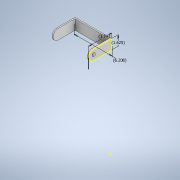
# Autodesk Inventor part: small side peice
Saved by Autodesk Inventor 2021 (Build 250183000, 183)
## iProperties
Created: 2021-08-21
Part Number: small side peice
Material: Generic
Document SubType Name: Modeling
Designer: newic
Density: 1 g/cm^3
Appearance: Default
Author: newic
Autodesk Inventor part; units mm, degrees
ref_plane "YZ Plane" through (0, 0, 0) normal (1, 0, 0) x (0, 1, 0)
ref_plane "XZ Plane" through (0, 0, 0) normal (0, 1, 0) x (-1, 0, 0)
ref_plane "XY Plane" through (0, 0, 0) normal (0, 0, 1) x (1, 0, 0)
sketch "Sketch1" plane through (0, 0, 0) normal (1, 0, 0) x (0, 1, 0)
  line L0 (920.75, 0) -> (0, 0)
  line L1 (0, 0) -> (920.75, 0)
  line L2 (-297.6389, 409.8513) -> (2710.7909, 409.8513) construction
  line L3 (2710.7909, 409.8513) -> (2710.7909, -1716.9746) construction
  line L4 (2710.7909, -1716.9746) -> (-297.6389, -1716.9746) construction
  line L5 (-297.6389, -1716.9746) -> (-297.6389, 409.8513) construction
  line L6 (0, 0) -> (920.75, 0)
  line L7 (920.75, 0) -> (920.75, 100.33)
  line L8 (0, 100.33) -> (920.75, 100.33)
  line L9 (0, 0) -> (0, 100.33)
  line L10 (0, 100.33) -> (0, 120.65)
  line L11 (0, 120.65) -> (920.75, 120.65)
  line L12 (920.75, 120.65) -> (920.75, 100.33)
  line L13 (0, 120.65) -> (0, 196.85)
  line L14 (920.75, 196.85) -> (920.75, 120.65)
  line L15 (477.9962, 0) -> (477.9962, -13.97)
  line L16 (477.9962, -13.97) -> (434.8162, -13.97)
  line L17 (434.8162, -13.97) -> (434.8162, 0)
  line L18 (133.294, 0) -> (133.294, -13.97)
  line L19 (133.294, -13.97) -> (90.114, -13.97)
  line L20 (90.114, -13.97) -> (90.114, 0)
  line L21 (769.0257, 0) -> (769.0257, -13.97)
  line L22 (769.0257, -13.97) -> (812.2057, -13.97)
  line L23 (812.2057, -13.97) -> (812.2057, 0)
  line L24 (434.8162, -13.97) -> (477.9962, -13.97)
  line L25 (769.0257, -13.97) -> (812.2057, -13.97)
  line L26 (90.114, -13.97) -> (133.294, -13.97)
  line L27 (90.114, -13.97) -> (111.704, -13.97)
  line L28 (111.704, -13.97) -> (100.909, -13.97)
  line L29 (100.909, -13.97) -> (122.499, -13.97)
  line L30 (122.499, -13.97) -> (122.499, -33.02)
  line L31 (122.499, -33.02) -> (100.909, -33.02)
  line L32 (100.909, -33.02) -> (100.909, -13.97)
  line L33 (434.8162, -13.97) -> (456.4062, -13.97)
  line L34 (456.4062, -13.97) -> (445.6112, -13.97)
  line L35 (445.6112, -13.97) -> (467.2012, -13.97)
  line L36 (467.2012, -13.97) -> (467.2012, -33.02)
  line L37 (467.2012, -33.02) -> (445.6112, -33.02)
  line L38 (445.6112, -33.02) -> (445.6112, -13.97)
  line L39 (769.0257, -13.97) -> (790.6157, -13.97)
  line L40 (790.6157, -13.97) -> (779.8207, -13.97)
  line L41 (779.8207, -13.97) -> (801.4107, -13.97)
  line L42 (801.4107, -13.97) -> (801.4107, -33.02)
  line L43 (801.4107, -33.02) -> (779.8207, -33.02)
  line L44 (779.8207, -33.02) -> (779.8207, -13.97)
  line L45 (434.8162, 0) -> (413.2262, 0)
  line L46 (413.2262, 0) -> (413.2262, -11.43)
  line L47 (413.2262, -11.43) -> (371.9512, -11.43)
  line L48 (371.9512, -11.43) -> (371.9512, 64.77)
  arc A0 (413.2262, 72.0379) -> (371.9512, 72.0379) centre (392.5887, 68.404) ccw
  line L49 (413.2262, 0) -> (413.2262, 64.77)
  line L50 (371.9512, 64.77) -> (371.9512, 72.0379)
  line L51 (413.2262, 64.77) -> (413.2262, 72.0379)
  line L52 (434.8162, -13.97) -> (434.8162, 202.565)
  line L53 (477.9962, -13.97) -> (477.9962, 202.565)
  line L54 (769.0257, -13.97) -> (769.0257, 202.565)
  line L55 (812.2057, -13.97) -> (812.2057, 202.565)
  line L56 (812.2057, 202.565) -> (769.0257, 202.565)
  line L57 (477.9962, 202.565) -> (434.8162, 202.565)
  line L58 (133.294, -13.97) -> (133.294, 182.245)
  line L59 (90.114, -13.97) -> (90.114, 182.245)
  line L60 (90.114, 182.245) -> (133.294, 182.245)
  line L61 (67.3834, 182.245) -> (164.6776, 182.245)
  line L62 (413.2262, 202.565) -> (508.4774, 202.565)
  line L63 (745.5808, 202.565) -> (847.3717, 202.565)
  line L64 (67.3834, 161.925) -> (164.6776, 161.925)
  line L65 (413.2262, 182.245) -> (508.4774, 182.245)
  line L66 (745.5808, 182.245) -> (847.3717, 182.245)
  line L67 (133.294, -13.97) -> (133.294, 78.74)
  line L68 (133.294, 78.74) -> (434.8162, 78.74)
  line L69 (133.294, -13.97) -> (133.294, 26.67)
  line L70 (133.294, 26.67) -> (371.9512, 26.67)
  line L71 (133.294, 26.67) -> (298.394, 26.67)
  line L72 (298.394, 26.67) -> (317.7759, 78.74)
  line L73 (133.294, 78.74) -> (133.294, 59.055)
  line L74 (133.294, 59.055) -> (310.4486, 59.055)
  line L75 (371.9512, 0) -> (371.9512, -5.715)
  line L76 (371.9512, -5.715) -> (413.2262, -5.715)
  dimension "d0" = 920.75
  dimension "d1" = 20.32
  dimension "d2" = 76.2
  dimension "d3" = 13.97
  dimension "d4" = 43.18
  dimension "d5" = 13.97
  dimension "d6" = 43.18
  dimension "d7" = 13.97
  dimension "d8" = 13.97
  dimension "d9" = 43.18
  dimension "d10" = 21.59
  dimension "d11" = 19.05
  dimension "d12" = 21.59
  dimension "d13" = 19.05
  dimension "d14" = 21.59
  dimension "d15" = 19.05
  dimension "d16" = 21.59
  dimension "d17" = 11.43
  dimension "d18" = 41.275
  dimension "d19" = 76.2
  dimension "d20" = 20.955
  dimension "d21" = 216.535
  dimension "d22" = 216.535
  dimension "d23" = 216.535
  dimension "d24" = 216.535
  dimension "d25" = 196.215
  dimension "d26" = 20.32
  dimension "d27" = 20.32
  dimension "d28" = 20.32
  dimension "d29" = 92.71
  dimension "d30" = 40.64
  dimension "d31" = 165.1
  dimension "d32" = 19.685
  constraints: 144 end point, 14 perpendicular, 13 point on line, 12 horizontal, 11 vertical, 10 equal length, 8 midpoint, 2 point on circle, 1 centre point, 13 other
  measures "d0" distance of L0.start L0.end
  measures "d1" distance of L8.start L10.end
  measures "d2" distance of L10.end L13.end
  measures "d3" distance of L15.start L15.end
  measures "d4" distance of L15.end L16.end
  measures "d5" distance of L18.start L18.end
  measures "d6" distance of L18.end L19.end
  measures "d7" distance of L19.end L20.end
  measures "d8" distance of L21.start L21.end
  measures "d9" distance of L21.end L22.end
  measures "d10" distance of L30.end L31.end
  measures "d11" distance of L29.end L30.end
  measures "d12" distance of L36.end L37.end
  measures "d13" distance of L35.end L36.end
  measures "d14" distance of L42.end L43.end
  measures "d15" distance of L41.end L42.end
  measures "d16" distance of L17.end L45.end
  measures "d17" distance of L45.end L46.end
  measures "d18" distance of L46.end L47.end
  measures "d19" distance of L47.end L48.end
  measures "d20" radius of A0
  measures "d21" distance of L16.end L52.end
  measures "d22" distance of L24.end L53.end
  measures "d23" distance of L21.end L54.end
  measures "d24" distance of L25.end L55.end
  measures "d25" distance of L26.end L58.end
  measures "d26" distance between parallel lines of L61 L64
  measures "d27" distance between parallel lines of L62 L65
  measures "d28" distance between parallel lines of L63 L66
  measures "d29" distance of L26.end L67.end
  measures "d30" distance of L26.end L69.end
  measures "d31" distance of L69.end L71.end
  measures "d32" distance of L67.end L73.end
extrude "Extrusion1" add sketch "Sketch1" along normal blind 5.715 and the other way blind 145.415 contours L46 L76 L48 L0 | L0 L48 L50 A0 L68 L51 L49 | L68 A0
sketch "Sketch2" plane through (-145.415, 413.2262, 72.0379) normal (0, 1, 0) x (1, 0, 0)
  line L0 (0, 0) -> (151.13, 0) projected
  line L1 (151.13, 77.7529) -> (151.13, 0) projected
  line L2 (0, 77.7529) -> (151.13, 77.7529) projected
  line L3 (0, 0) -> (0, 77.7529) projected
  line L4 (144.145, 70.7679) -> (144.145, 6.985)
  line L5 (144.145, 6.985) -> (6.985, 6.985)
  line L6 (6.985, 6.985) -> (6.985, 70.7679)
  line L7 (6.985, 70.7679) -> (144.145, 70.7679)
  line L8 (146.05, 72.6729) -> (146.05, 5.08)
  line L9 (146.05, 5.08) -> (5.08, 5.08)
  line L10 (5.08, 5.08) -> (5.08, 72.6729)
  line L11 (5.08, 72.6729) -> (146.05, 72.6729)
  line L12 (146.05, 5.08) -> (146.05, -20.9448)
  line L13 (146.05, 5.08) -> (172.0748, 5.08) construction
  line L14 (5.08, 5.08) -> (5.08, -29.2393)
  line L15 (5.08, -29.2393) -> (146.05, -20.9448)
  point P0 (145.415, 72.0379)
  dimension "d39" = 6.985
  dimension "d40" = 1.905
  dimension "d41" = 90
  constraints: 24 end point, 1 horizontal, 1 perpendicular, 1 vertical, 6 other
  measures "d39" distance between parallel lines of L2 L7
  measures "d40" distance between parallel lines of L7 L11
  measures "d41" angle of L12 L13
extrude "Extrusion2" cut sketch "Sketch2" against normal through all contours L14 L9 L12 L0 | L0 L12 L15 L14 | L10 L11 L8 L9 | L4 L5 L6 L7
sketch "Sketch3" plane through (5.715, 0, 0) normal (1, 0, 0) x (0, 0, -1)
  arc A0 (-72.0379, 413.2262) -> (-72.0379, 371.9512) centre (-68.404, 392.5887) ccw projected
  circle A1 centre (-68.404, 392.5887) radius 6.6675
  point P0 (0, 0)
  dimension "d44" = 13.335
  constraints: 1 centre point, 1 coincident
  measures "d44" diameter of A1
sketch "Sketch4" plane through (-145.415, 0, 0) normal (-1, 0, 0) x (0, 0, 1)
  circle A0 centre (68.404, 392.5887) radius 6.6675 projected
  circle A1 centre (68.404, 392.5887) radius 6.6675
  point P0 (0, 0)
  constraints: 1 centre point, 1 coincident, 1 concentric
extrude "Extrusion3" add sketch "Sketch4" along normal blind 3.175
extrude "Extrusion4" add sketch "Sketch3" along normal blind 3.175
fillet "Fillet1" radius 2.286 2 edges at (8.89, 392.5887, 75.0715) (-148.59, 392.5887, 61.7365)
sketch "Sketch5" plane through (5.715, 0, 0) normal (1, 0, 0) x (0, 0, -1)
  arc A0 (-72.0379, 413.2262) -> (-72.0379, 371.9512) centre (-68.404, 392.5887) ccw projected
  line L0 (-89.359, 392.5887) -> (-89.359, 351.6635)
  line L1 (5.715, 371.9512) -> (5.715, 413.2262) projected
  line L2 (-72.0379, 371.9512) -> (5.715, 371.9512) projected
  line L3 (5.715, 413.2262) -> (-72.0379, 413.2262) projected
  point P0 (0, 0)
  dimension "d50" = 95.0739
  dimension "d51" = 41.275
  constraints: 2 end point, 1 point on circle, 1 tangent, 1 vertical
  measures "d50" distance from line of L1 L0.start
  measures "d51" distance between parallel lines of L2 L3
sketch "Sketch6" plane through (5.715, 413.2262, -5.715) normal (0, 0, -1) x (-1, 0, 0)
  line L0 (154.305, -16.256) -> (154.305, -25.019) projected
  line L1 (-3.175, -25.019) -> (-3.175, -16.256) projected
  point P0 (5.715, -413.2262)
  dimension "d52" = 157.48
  measures "d52" distance between parallel lines of L0 L1
body "Solid1"
